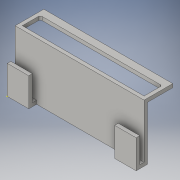
# Autodesk Inventor part: Handles
Saved by Autodesk Inventor 2016 (Build 200138000, 138)
## iProperties
Created: 2017-03-11
Part Number: Handles
Material: Generic
Document SubType Name: Modeling
Designer: RoboticsUser
Density: 1 g/cm^3
Appearance: Default
Author: RoboticsUser
Autodesk Inventor part; units mm, degrees
ref_plane "YZ Plane" through (0, 0, 0) normal (1, 0, 0) x (0, 1, 0)
ref_plane "XZ Plane" through (0, 0, 0) normal (0, 1, 0) x (-1, 0, 0)
ref_plane "XY Plane" through (0, 0, 0) normal (0, 0, 1) x (1, 0, 0)
sketch "Sketch1" plane through (0, 0, 0) normal (1, 0, 0) x (0, 1, 0)
  line L0 (0, 0) -> (101.6, 0)
  line L1 (101.6, 0) -> (101.6, -64.77)
  line L2 (101.6, -64.77) -> (0, -64.77)
  line L3 (0, -64.77) -> (0, 0)
  line L4 (101.6, -6.35) -> (6.35, -6.35)
  line L5 (6.35, -6.35) -> (6.35, -13.97)
  line L6 (6.35, -13.97) -> (101.6, -13.97)
  line L7 (101.6, -13.97) -> (101.6, -6.35)
  line L8 (0, -64.77) -> (95.25, -64.77)
  line L9 (95.25, -64.77) -> (95.25, -20.32)
  line L10 (95.25, -20.32) -> (0, -20.32)
  line L11 (0, -20.32) -> (0, -64.77)
  line L12 (101.6, 0) -> (50.8, 0)
  line L13 (50.8, 0) -> (50.8, -6.35)
  line L14 (50.8, -6.35) -> (101.6, -6.35)
  line L15 (101.6, -6.35) -> (101.6, 0)
  dimension "d0" = 101.6
  dimension "d1" = 64.77
  dimension "d2" = 95.25
  dimension "d3" = 7.62
  dimension "d4" = 6.35
  dimension "d5" = 95.25
  dimension "d6" = 44.45
  dimension "d7" = 50.8
  constraints: 32 end point, 8 parallel, 4 horizontal, 4 perpendicular, 2 point on line
  measures "d0" distance of L1.end L2.end
  measures "d1" distance of L0.end L1.end
  measures "d2" distance of L6.end L5.end
  measures "d3" distance of L5.end L4.end
  measures "d4" distance between parallel lines of L4 L0
  measures "d5" distance of L10.end L9.end
  measures "d6" distance of L9.end L8.end
  measures "d7" distance of L14.end L13.end
sketch "Sketch2" plane through (0, 0, 0) normal (1, 0, 0) x (0, 1, 0)
  point P0 (0, 0)
extrude "Extrusion1" add sketch "Sketch1" along normal blind 228.6 contours L0 L13 L4 L5 L6 L1 L2 L9 L10 L3
sketch "Sketch3" plane through (0, 101.6, -13.97) normal (0, 1, 0) x (1, 0, 0)
  line L0 (0, 0) -> (228.6, 0) projected
  line L1 (0, 50.8) -> (228.6, 50.8) projected
  line L2 (0, -7.62) -> (228.6, -7.62) projected
  line L3 (228.6, -13.97) -> (0, -13.97) projected
  line L4 (0, 50.8) -> (0, 0) projected
  line L5 (228.6, 50.8) -> (228.6, 0) projected
  line L6 (228.6, 0) -> (228.6, -7.62) projected
  line L7 (228.6, -7.62) -> (228.6, -13.97) projected
  line L8 (0, -13.97) -> (0, -7.62) projected
  line L9 (0, -7.62) -> (0, 0) projected
  line L10 (0, 6.35) -> (228.6, 6.35) projected
  line L11 (6.35, 6.35) -> (222.25, 6.35)
  line L12 (222.25, 6.35) -> (222.25, 34.925)
  line L13 (219.075, 38.1) -> (9.525, 38.1)
  line L14 (6.35, 34.925) -> (6.35, 6.35)
  arc A0 (9.525, 38.1) -> (6.35, 34.925) centre (9.525, 34.925) ccw
  arc A1 (222.25, 34.925) -> (219.075, 38.1) centre (219.075, 34.925) ccw
  point P0 (222.25, 38.1)
  point P1 (6.35, 38.1)
  dimension "d10" = 215.9
  dimension "d11" = 31.75
  dimension "d12" = 6.35
  dimension "d13" = 3.175
  dimension "d14" = 3.175
  constraints: 8 end point, 5 point on line, 4 point on circle, 4 tangent, 2 centre point, 2 parallel, 1 horizontal, 1 perpendicular
  measures "d10" distance of point (6.35, 38.1) point (222.25, 38.1)
  measures "d11" distance of point (222.25, 38.1) L11.end
  measures "d12" distance between parallel lines of L14 L4
  measures "d13" radius of A0
  measures "d14" radius of A1
extrude "Extrusion2" cut sketch "Sketch3" against normal blind 228.6 contours L14 A0 L13 A1 L12 L10
sketch "Sketch4" plane through (0, 101.6, -13.97) normal (0, 1, 0) x (1, 0, 0)
  line L0 (0, -13.97) -> (0, -7.62) projected
  line L1 (228.6, -13.97) -> (0, -13.97) projected
  line L2 (228.6, -7.62) -> (228.6, -13.97) projected
  line L3 (0, -7.62) -> (228.6, -7.62) projected
  line L4 (6.0709, -13.97) -> (221.9709, -13.97)
  line L5 (221.9709, 0) -> (6.0709, 0)
  line L6 (38.1, -13.97) -> (190.5, -13.97)
  line L7 (190.5, -13.97) -> (190.5, 0)
  line L8 (190.5, 0) -> (38.1, 0)
  line L9 (38.1, 0) -> (38.1, -13.97)
  dimension "d19" = 215.9
  dimension "d23" = 152.4
  dimension "d24" = 13.97
  dimension "d25" = 38.1
  constraints: 12 end point, 3 parallel, 2 horizontal, 2 point on line, 1 perpendicular
  measures "d19" distance of L5.end L5.start
  measures "d23" distance of L8.end L7.end
  measures "d24" distance of L6.end L7.end
  measures "d25" distance between parallel lines of L0 L9
extrude "Extrusion3" cut sketch "Sketch4" against normal blind 228.6 contours L9 L5 L7 L3 | L3 L7 L1 L9
body "Solid1"
